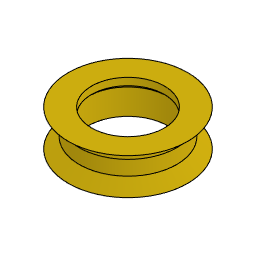
roller (Autodesk Fusion 360 design; units mm, degrees)
Autodesk Fusion 360 part; units mm, degrees
note: some values were not read from the file. Set by a fixed rule: which sketch regions a step uses.
sketch "Sketch1" plane through (0, 0, 0) normal (0, 1, 0) x (1, 0, 0)
  line L0 (0, 0) -> (11, 0)
  line L1 (11, 0) -> (11, -10)
  line L2 (11, -10) -> (0, -10)
  line L3 (0, -10) -> (0, 0)
  line L4 (11, -10) -> (16.4, -10)
  line L5 (16.4, -10) -> (13.4, -7)
  line L6 (13.4, -7) -> (13.4, -3)
  line L7 (13.4, -3) -> (16.4, 0)
  line L8 (16.4, 0) -> (11, 0)
  line L9 (11, -7) -> (10, -7)
  line L10 (10, -7) -> (10, -10)
  line L11 (11, -7) -> (10, -8)
  line L12 (11, -7) -> (12.3815, -7) construction
  dimension "d1" = 11
  dimension "d2" = 10
  dimension "d3" = 2.4
  dimension "d4" = 3
  dimension "d5" = 45
  dimension "d10" = 3
  dimension "d11" = 1
  dimension "d12" = 135
  constraint horizontal L0
  constraint vertical L1
  constraint horizontal L2
  constraint vertical L3
  constraint coincident L0.start L3.end
  constraint perpendicular L1 L4
  constraint perpendicular L4 L6
  constraint horizontal L8
  constraint vertical L4.end L7.end
  constraint equal L5 L7
  constraint coincident L1 L9.start
  constraint perpendicular L1 L9
  constraint coincident L2 L10.end
  constraint perpendicular L2 L10
  constraint horizontal L12
  constraint coincident L10 L11.end
  measures "d1" distance of L0.start L0.end
  measures "d2" distance of L0.start L2.end
  measures "d3" distance of L1 L6
  measures "d4" distance of L4.end L6
  measures "d5" angle of L4 L5
  measures "d10" distance of L9.end L10.end
  measures "d11" distance of L1 L10
  measures "d12" angle of L11 L12
revolve "Revolve1" add sketch "Sketch1" angle 360 about axis through (0, 0, 1.75) along (0, 0, 1) contours L1 L4 L5 L6 L7 L8 | L1 L2 L10 L11
equation "d5 = 45 °"
equation "d12 = 135 °"
